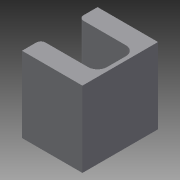
# Autodesk Inventor part: Hook0
Saved by Autodesk Inventor 2015 (Build 190159000, 159)
## iProperties
Created: 2015-01-20
Part Number: Hook0
Material: Generic
Document SubType Name: Modeling
Designer: christopherroche
Density: 1 g/cm^3
Appearance: Default
Author: christopherroche
Autodesk Inventor part; units mm, degrees
ref_plane "YZ Plane" through (0, 0, 0) normal (1, 0, 0) x (0, 1, 0)
ref_plane "XZ Plane" through (0, 0, 0) normal (0, 1, 0) x (-1, 0, 0)
ref_plane "XY Plane" through (0, 0, 0) normal (0, 0, 1) x (1, 0, 0)
sketch "Sketch1" plane through (0, 0, 0) normal (0, 1, 0) x (-1, 0, 0)
  line L0 (0, 0) -> (0, 25.4)
  line L1 (40.64, 25.4) -> (40.64, 12.7)
  line L2 (40.64, 12.7) -> (2.54, 12.7)
  line L3 (0, 25.4) -> (40.64, 25.4)
  line L4 (0, 0) -> (0, -25.4)
  line L5 (0, -25.4) -> (40.64, -25.4)
  line L6 (40.64, -25.4) -> (40.64, -12.7)
  line L7 (40.64, -12.7) -> (2.54, -12.7)
  line L8 (2.54, -12.7) -> (2.54, 12.7)
  dimension "d2" = 38.1
  dimension "d5" = 25.4
  dimension "d8" = 2.54
  dimension "d9" = 38.1
  dimension "d10" = 12.7
  dimension "d11" = 12.7
  dimension "d12" = 25.4
  constraints: 18 end point, 4 vertical, 2 perpendicular, 1 collinear, 1 horizontal, 1 parallel
  measures "d2" distance of L1.end L2.end
  measures "d5" distance of L0.start L0.end
  measures "d8" distance between parallel lines of L4 L8
  measures "d9" distance of L6.end L7.end
  measures "d10" distance of L1.start L1.end
  measures "d11" distance of L5.end L6.end
  measures "d12" distance of L7.end L2.end
extrude "Extrusion1" add sketch "Sketch1" along normal blind 50.8
fillet "Fillet1" radius 6.35 1 edges at (-2.54, 25.4, -12.7)
fillet "Fillet2" radius 6.35 1 edges at (-2.54, 25.4, 12.7)
fillet "Fillet3" radius 3.175 1 edges at (-40.64, 25.4, -12.7)
fillet "Fillet4" radius 3.175 1 edges at (-40.64, 25.4, 12.7)
body "Solid1"
